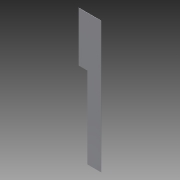
# Autodesk Inventor part: Mi
Saved by Autodesk Inventor 2014 SP1 (Build 180222100, 222)
## iProperties
Created: 2015-03-28
Part Number: Mi
Material: LCP Plastic
Document SubType Name: Modeling
Designer: tuleu
Density: 1.626 g/cm^3
Appearance: PVC - White
Author: tuleu
Autodesk Inventor part; units mm, degrees
ref_plane "YZ Plane" through (0, 0, 0) normal (1, 0, 0) x (0, 1, 0)
ref_plane "XZ Plane" through (0, 0, 0) normal (0, 1, 0) x (-1, 0, 0)
ref_plane "XY Plane" through (0, 0, 0) normal (0, 0, 1) x (1, 0, 0)
sketch "Sketch1" plane through (0, 0, 0) normal (0, 1, 0) x (-1, 0, 0)
  line L0 (20, -525) -> (-90, -525)
  line L1 (-90, 525) -> (90, 525)
  line L2 (0, 525) -> (0, -525)
  line L3 (20, -525) -> (20, 125)
  line L4 (20, 125) -> (90, 125)
  line L5 (90, 525) -> (90, 125)
  line L6 (20, 0) -> (-90, 0)
  line L7 (-90, 525) -> (-90, -525)
  point P0 (0, 0)
  dimension "d6" = 1050
  dimension "d7" = 180
  dimension "d8" = 70
  dimension "d10" = 650
  constraints: 16 end point, 3 midpoint, 3 perpendicular, 3 point on line, 2 parallel, 1 horizontal, 1 other
  measures "d6" distance between parallel lines of L1 L0
  measures "d7" distance of L1.start L1.end
  measures "d8" distance between parallel lines of L3 L5
  measures "d10" distance between parallel lines of L0 L4
extrude "Extrusion1" add sketch "Sketch1" along normal blind 2
body "Solid1"
